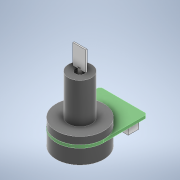
# Autodesk Inventor part: AT 25-5246
Saved by Autodesk Inventor 2021 (Build 250183000, 183)
## iProperties
Created: 2021-04-06
Part Number: AT 25-5246
Material: ABS Plastic
Document SubType Name: Modeling
Designer: Andrew
Density: 1.06 g/cm^3
Appearance: Smooth - White
Author: Andrew
Autodesk Inventor part; units mm, degrees
ref_plane "YZ Plane" through (0, 0, 0) normal (1, 0, 0) x (0, 1, 0)
ref_plane "XZ Plane" through (0, 0, 0) normal (0, 1, 0) x (-1, 0, 0)
ref_plane "XY Plane" through (0, 0, 0) normal (0, 0, 1) x (1, 0, 0)
sketch "Sketch1" plane through (0, 0, 0) normal (0, 0, 1) x (1, 0, 0)
  line L0 (0, 0) -> (13, 0)
  line L1 (13, 0) -> (13, 8)
  line L2 (13, 8) -> (0, 8)
  line L3 (0, 8) -> (0, 0)
  line L4 (12, 9.57) -> (13, 9.57)
  line L5 (13, 9.57) -> (13, 13.57)
  line L6 (13, 13.57) -> (6.35, 13.57)
  line L7 (6.35, 13.57) -> (6.35, 35.57)
  line L8 (6.35, 35.57) -> (2.5, 35.57)
  line L9 (2.5, 35.57) -> (2.5, 34.57)
  line L10 (2.5, 34.57) -> (5.35, 34.57)
  line L11 (5.35, 34.57) -> (5.35, 12.57)
  line L12 (5.35, 12.57) -> (12, 12.57)
  line L13 (12, 12.57) -> (12, 9.57)
  line L14 (0.875, 22.57) -> (0, 22.57)
  line L15 (0, 22.57) -> (0, 37.57)
  line L16 (0, 37.57) -> (0.875, 37.57)
  line L17 (0.875, 37.57) -> (0.875, 22.57)
  line L18 (-3.5, 36.57) -> (3.5, 36.57)
  line L19 (3.5, 36.57) -> (3.5, 47.57)
  line L20 (3.5, 47.57) -> (-3.5, 47.57)
  line L21 (-3.5, 47.57) -> (-3.5, 36.57)
  line L22 (-3.5, 36.57) -> (3.5, 47.57) construction
  line L23 (3.5, 36.57) -> (-3.5, 47.57) construction
  point P0 (0, 42.07)
  point P1 (0, 42.07)
  dimension "d0" = 8
  dimension "d1" = 4
  dimension "d2" = 13
  dimension "d3" = 1.57
  dimension "d4" = 22
  dimension "d6" = 1
  dimension "d7" = 1
  dimension "d8" = 1
  dimension "d9" = 1
  dimension "d10" = 6.35
  dimension "d11" = 0.875
  dimension "d12" = 2.5
  dimension "d13" = 2
  dimension "d14" = 15
  dimension "d15" = 11
  dimension "d16" = 7
  dimension "d17" = 1
  constraints: 48 end point, 13 perpendicular, 4 horizontal, 4 parallel, 3 midpoint, 3 point on line, 1 collinear
  measures "d0" distance of L0.end L1.end
  measures "d1" distance of L4.end L5.end
  measures "d2" distance of L0.start L0.end
  measures "d3" distance between parallel lines of L2 L4
  measures "d4" distance of L6.end L7.end
  measures "d6" distance between parallel lines of L10 L8
  measures "d7" distance between parallel lines of L7 L11
  measures "d8" distance between parallel lines of L6 L12
  measures "d9" distance between parallel lines of L5 L13
  measures "d10" distance between parallel lines of L3 L7
  measures "d11" distance between parallel lines of L15 L17
  measures "d12" distance between parallel lines of L3 L9
  measures "d13" distance between parallel lines of L8 L16
  measures "d14" distance of L14.end L15.end
  measures "d15" distance of L20.end L18.start
  measures "d16" distance of L19.end L20.end
  measures "d17" distance between parallel lines of L8 L18
revolve "Revolution1" add sketch "Sketch1" angle 360 about axis through (0, 8, 0) along (0, -1, 0) contours L3 L2 L1 L0 | L13 L12 L11 L10 L9 L8 L7 L6 L5 L4
revolve "Revolution2" add sketch "Sketch1" angle 360 about axis through (0, 22.57, 0) along (0, 1, 0) separate body contours L14 L15 L18 L17 | L18 L15 L16 L17
extrude "Extrusion1" add sketch "Sketch1" against normal mid plane 0.75 separate body contours L18 L15 L16 L17 | L17 L16 L15 L18 L21 L20 L19
sketch "Sketch2" plane through (0, 0, 0) normal (0, 1, 0) x (-1, 0, 0)
  circle A0 centre (0, 0) radius 0.875 projected
  arc A1 (13, 0) -> (-13, 0) centre (0, 0) ccw
  line L0 (-13, 0) -> (-13, -24)
  line L1 (-13, -24) -> (13, -24)
  line L2 (13, -24) -> (13, 0)
  line L3 (-8.75, -23.5) -> (8.75, -23.5)
  line L4 (8.75, -23.5) -> (8.75, -17.75)
  line L5 (8.75, -17.75) -> (-8.75, -17.75)
  line L6 (-8.75, -17.75) -> (-8.75, -23.5)
  line L7 (-8.75, -23.5) -> (8.75, -17.75) construction
  line L8 (8.75, -23.5) -> (-8.75, -17.75) construction
  point P0 (0, 0)
  point P1 (-13, 0)
  point P2 (-13, 0)
  point P3 (-13, 0)
  point P4 (0, -20.625)
  point P5 (0, -20.625)
  point P6 (0, -24)
  dimension "d23" = 37
  dimension "d24" = 17.5
  dimension "d25" = 5.75
  dimension "d26" = 0.5
  constraints: 18 end point, 4 midpoint, 3 perpendicular, 3 point on circle, 2 parallel, 2 tangent, 1 centre point, 1 coincident, 1 horizontal, 1 vertical, 1 vertical alignment
  measures "d24" distance of L4.end L5.end
  measures "d25" distance of L3.end L4.end
  measures "d26" distance between parallel lines of L1 L3
extrude "Extrusion2" add sketch "Sketch2" along normal up to surface (1.57 mm away) from surface at 8 separate body contours L2 L1 L0 A1 | L6 L5 L4 L3
extrude "Extrusion3" add sketch "Sketch2" against normal blind 7.5 from surface at 8 separate body contours L6 L5 L4 L3
chamfer "Chamfer1" distance 1 angle 45 2 edges at (-13, 8.785, -24) (13, 8.785, -24)
body "Solid1"
body "Solid2"
body "Solid3"
body "Solid4"
body "Solid5"
